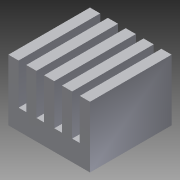
# Autodesk Inventor part: SmallHeatsink
Saved by Autodesk Inventor 2014 (Build 180170000, 170)
## iProperties
Created: 2015-11-06
Part Number: SmallHeatsink
Material: Generic
Document SubType Name: Modeling
Designer: Owner
Density: 1 g/cm^3
Appearance: Aluminum - Flat
Author: Owner
Autodesk Inventor part; units mm, degrees
ref_plane "YZ Plane" through (0, 0, 0) normal (1, 0, 0) x (0, 1, 0)
ref_plane "XZ Plane" through (0, 0, 0) normal (0, 1, 0) x (-1, 0, 0)
ref_plane "XY Plane" through (0, 0, 0) normal (0, 0, 1) x (1, 0, 0)
sketch "Sketch1" plane through (0, 0, 0) normal (0, 0, 1) x (1, 0, 0)
  line L0 (-4.5765, 3.9949) -> (3.4235, 3.9949)
  line L1 (3.4235, 3.9949) -> (3.4235, -2.0051)
  line L2 (3.4235, -2.0051) -> (-4.5765, -2.0051)
  line L3 (-4.5765, -2.0051) -> (-4.5765, 3.9949)
  line L4 (-4.5765, -0.0051) -> (3.4235, -0.0051)
  line L5 (-3.5765, 3.9949) -> (-2.8265, 3.9949)
  line L6 (-2.8265, 3.9949) -> (-2.8265, -0.0051)
  line L7 (-2.8265, -0.0051) -> (-3.5765, -0.0051)
  line L8 (-3.5765, -0.0051) -> (-3.5765, 3.9949)
  line L9 (-1.8265, 3.9949) -> (-1.0765, 3.9949)
  line L10 (-1.0765, 3.9949) -> (-1.0765, -0.0051)
  line L11 (-1.0765, -0.0051) -> (-1.8265, -0.0051)
  line L12 (-1.8265, -0.0051) -> (-1.8265, 3.9949)
  line L13 (1.6735, 3.9949) -> (2.4235, 3.9949)
  line L14 (2.4235, 3.9949) -> (2.4235, -0.0051)
  line L15 (2.4235, -0.0051) -> (1.6735, -0.0051)
  line L16 (1.6735, -0.0051) -> (1.6735, 3.9949)
  line L17 (-0.0765, 3.9949) -> (0.6735, 3.9949)
  line L18 (0.6735, 3.9949) -> (0.6735, -0.0051)
  line L19 (0.6735, -0.0051) -> (-0.0765, -0.0051)
  line L20 (-0.0765, -0.0051) -> (-0.0765, 3.9949)
  point P0 (0, 0)
  dimension "d0" = 6
  dimension "d1" = 8
  dimension "d2" = 2
  dimension "d3" = 1
  dimension "d4" = 1
  dimension "d5" = 1
  dimension "d6" = 1
  dimension "d7" = 1
  dimension "d8" = 0.75
  dimension "d9" = 0.75
  dimension "d10" = 0.75
  constraints: 42 end point, 10 parallel, 10 point on line, 6 perpendicular, 5 horizontal
  measures "d0" distance of L2.end L0.start
  measures "d1" distance of L1.end L2.end
  measures "d2" distance between parallel lines of L2 L4
  measures "d3" distance between parallel lines of L3 L8
  measures "d4" distance between parallel lines of L12 L6
  measures "d5" distance between parallel lines of L20 L10
  measures "d6" distance between parallel lines of L16 L18
  measures "d7" distance between parallel lines of L1 L14
  measures "d8" distance between parallel lines of L8 L6
  measures "d9" distance between parallel lines of L10 L12
  measures "d10" distance between parallel lines of L18 L20
extrude "Extrusion1" add sketch "Sketch1" along normal blind 8 contours L0 L8 L4 L3 | L4 L1 L2 L3 | L0 L12 L4 L6 | L0 L20 L4 L10 | L4 L14 L0 L1 | L0 L16 L4 L18
body "Solid1"
